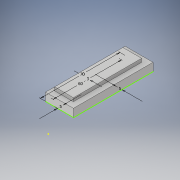
# Autodesk Inventor part: LCD-Display
Saved by Autodesk Inventor 2019.5 (Build 235369000, 369)
## iProperties
Created: 2021-10-01
Part Number: LCD-Display
Material: Generisch
Document SubType Name: Modeling
Designer: mritt
Density: 1 g/cm^3
Appearance: Vorgabe
Author: mritt
Autodesk Inventor part; units mm, degrees
ref_plane "YZ Plane" through (0, 0, 0) normal (1, 0, 0) x (0, 1, 0)
ref_plane "XZ Plane" through (0, 0, 0) normal (0, 1, 0) x (-1, 0, 0)
ref_plane "XY Plane" through (0, 0, 0) normal (0, 0, 1) x (1, 0, 0)
sketch "Skizze1" plane through (0, 0, 0) normal (0, 1, 0) x (-1, 0, 0)
  line L0 (26.173, -23.607) -> (1.6422, -23.607)
  line L1 (1.6422, -23.607) -> (1.6422, -93.607)
  line L2 (1.6422, -93.607) -> (26.173, -93.607)
  line L3 (26.173, -93.607) -> (26.173, -23.607)
  line L4 (23.173, -28.607) -> (6.6422, -28.607)
  line L5 (6.6422, -28.607) -> (6.6422, -88.607)
  line L6 (6.6422, -88.607) -> (23.173, -88.607)
  line L7 (23.173, -88.607) -> (23.173, -28.607)
  point P0 (0, 0)
  dimension "d0" = 70
  dimension "d1" = 60
  dimension "d2" = 5
  dimension "d3" = 5
  dimension "d4" = 3
  constraints: 16 end point, 4 parallel, 2 horizontal, 2 perpendicular
  measures "d0" distance of L2.end L0.start
  measures "d1" distance of L6.end L4.start
  measures "d2" distance between parallel lines of L4 L0
  measures "d3" distance between parallel lines of L5 L1
  measures "d4" distance between parallel lines of L7 L3
extrude "Extrusion1" add sketch "Skizze1" along normal blind 7
extrude "Extrusion2" add sketch "Skizze1" along normal blind 10 contours L7 L6 L5 L4
